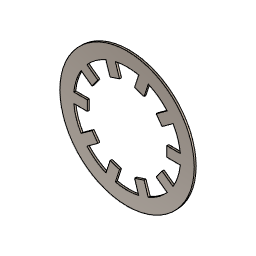
Inductive_Proximity_Washer (Autodesk Fusion 360 design; units mm, degrees)
Autodesk Fusion 360 part; units mm, degrees
sketch "Sketch1" plane through (0, 0, 0) normal (0, 1, 0) x (1, 0, 0)
  circle A0 centre (0, 0) radius 10.75
  circle A1 centre (0, 0) radius 8.55
  line L0 (-6.35, 0.8) -> (-6.35, -0.8)
  line L1 (-8.5125, 0.8) -> (-6.35, 0.8)
  line L2 (-6.35, -0.8) -> (-8.5125, -0.8)
  line L3 (-4.667, -4.3796) -> (-6.4165, -5.6507)
  line L4 (-7.357, -4.3563) -> (-5.6075, -3.0852)
  line L5 (-5.6075, -3.0852) -> (-4.667, -4.3796)
  line L6 (-1.2014, -6.2864) -> (-1.8697, -8.3431)
  line L7 (-3.3913, -7.8486) -> (-2.7231, -5.792)
  line L8 (-2.7231, -5.792) -> (-1.2014, -6.2864)
  line L9 (2.7231, -5.792) -> (3.3913, -7.8486)
  line L10 (1.8697, -8.3431) -> (1.2014, -6.2864)
  line L11 (1.2014, -6.2864) -> (2.7231, -5.792)
  line L12 (5.6075, -3.0852) -> (7.357, -4.3563)
  line L13 (6.4165, -5.6507) -> (4.667, -4.3796)
  line L14 (4.667, -4.3796) -> (5.6075, -3.0852)
  line L15 (6.35, 0.8) -> (8.5125, 0.8)
  line L16 (8.5125, -0.8) -> (6.35, -0.8)
  line L17 (6.35, -0.8) -> (6.35, 0.8)
  line L18 (4.667, 4.3796) -> (6.4165, 5.6507)
  line L19 (7.357, 4.3563) -> (5.6075, 3.0852)
  line L20 (5.6075, 3.0852) -> (4.667, 4.3796)
  line L21 (1.2014, 6.2864) -> (1.8697, 8.3431)
  line L22 (3.3913, 7.8486) -> (2.7231, 5.792)
  line L23 (2.7231, 5.792) -> (1.2014, 6.2864)
  line L24 (-2.7231, 5.792) -> (-3.3913, 7.8486)
  line L25 (-1.8697, 8.3431) -> (-1.2014, 6.2864)
  line L26 (-1.2014, 6.2864) -> (-2.7231, 5.792)
  line L27 (-5.6075, 3.0852) -> (-7.357, 4.3563)
  line L28 (-6.4165, 5.6507) -> (-4.667, 4.3796)
  line L29 (-4.667, 4.3796) -> (-5.6075, 3.0852)
  point P0 (-8.55, 0)
  point P1 (-8.55, 0)
  dimension "d1" = 21.5
  dimension "d2" = -2.2
  dimension "d8" = 360
  constraint coincident A0.centre A1.centre
  constraint horizontal L2
  constraint coincident P1 P0
  constraint coincident A1 L1.start
  constraint coincident A1 L2.end
  measures "d1" diameter of A0
extrude "Extrude1" add sketch "Sketch1" along normal blind 0.3 contours A0 | A1 L15 L16 L17 | A1 L18 L19 L20 | A1 L12 L13 L14 | A1 L21 L22 L23 | A1 L9 L10 L11 | A1 L24 L25 L26 | A1 L6 L7 L8 | A1 L27 L28 L29 | A1 L3 L4 L5 | A1 L0 L1 L2
